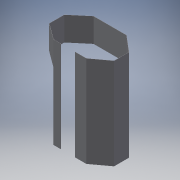
# Autodesk Inventor part: Main Cover
Saved by Autodesk Inventor 2016 (Build 200138000, 138)
## iProperties
Created: 2017-08-22
Part Number: Main Cover
Material: Generic
Document SubType Name: Modeling
Designer: m227586
Density: 1 g/cm^3
Appearance: Default
Author: m227586
Autodesk Inventor part; units mm, degrees
ref_plane "YZ Plane" through (0, 0, 0) normal (1, 0, 0) x (0, 1, 0)
ref_plane "XZ Plane" through (0, 0, 0) normal (0, 1, 0) x (-1, 0, 0)
sketch "Sketch2" plane through (0, 0, 0) normal (0, 0, 1) x (1, 0, 0)
  line L0 (7.8638, 351.0024) -> (-267.6362, 351.0024)
  line L1 (-267.6362, 351.0024) -> (-534, 125.5)
  line L2 (-534, 125.5) -> (-534, -125.5)
  line L3 (-534, -125.5) -> (-267.6362, -321.9976)
  line L4 (-267.6362, -321.9976) -> (7.8638, -321.9976)
  line L5 (7.8638, 351.0024) -> (7.8638, -321.9976) construction
  line L6 (-534, 0) -> (0, 0) construction
  line L7 (7.8638, 351.0024) -> (283.3638, 351.0024)
  line L8 (283.3638, 351.0024) -> (549.7276, 125.5)
  line L9 (549.7276, 125.5) -> (549.7276, -125.5)
  line L10 (549.7276, -125.5) -> (283.3638, -321.9976)
  line L11 (283.3638, -321.9976) -> (7.8638, -321.9976)
  dimension "d19" = 673
  dimension "d20" = 275.5
  dimension "d21" = 251
  dimension "d22" = 349
  dimension "d23" = 331
  dimension "d24" = 275.5
  dimension "d25" = 534
  constraints: 24 end point, 4 symmetric about line, 2 perpendicular, 2 vertical, 1 horizontal, 1 horizontal alignment, 1 midpoint
  measures "d19" distance of L0.start L4.end
  measures "d20" distance of L0.start L0.end
  measures "d21" distance of L1.end L2.end
  measures "d22" distance of L0.end L1.end
  measures "d23" distance of L2.end L3.end
  measures "d24" distance of L3.end L4.end
  measures "d25" distance of L6.start L6.end
ref_plane "Work Plane1" through (0, 0, 200) normal (0, 0, 1) x (1, 0, 0)
extrude "Extrusion1" add sketch "Sketch2" along normal blind 1306
shell "Shell2" thickness 3 removed faces 0
sketch "Sketch4" plane through (0, 0, 1306) normal (0, 0, 1) x (1, 0, 0)
  line L0 (-534, 125.5) -> (-267.6362, 351.0024)
  line L1 (-266.5368, 348.0024) -> (-531, 124.1091) projected
  line L2 (549.7276, 125.5) -> (283.3638, 351.0024) projected
  line L3 (-267.6362, 351.0024) -> (283.3638, 351.0024)
  line L4 (283.3638, 351.0024) -> (549.7276, 125.5)
  line L5 (546.7276, 124.1091) -> (282.2645, 348.0024) projected
  line L6 (283.3638, -321.9976) -> (549.7276, -125.5) projected
  line L7 (549.7276, 125.5) -> (549.7276, -125.5)
  line L8 (549.7276, -125.5) -> (283.3638, -321.9976)
  line L9 (-534, -125.5) -> (-267.6362, -321.9976) projected
  line L10 (283.3638, -321.9976) -> (-267.6362, -321.9976)
  line L11 (-534, 125.5) -> (-534, -125.5) projected
  line L12 (-267.6362, -321.9976) -> (-534, -125.5)
  line L13 (-534, -125.5) -> (-534, 125.5)
  line L14 (-531, 124.1091) -> (-531, -123.9851) projected
  point P0 (0, 0)
  constraints: 16 end point, 3 parallel, 2 collinear, 2 perpendicular, 1 horizontal
extrude "Extrusion2" cut sketch "Sketch4" against normal blind 3
sketch "Sketch5" plane through (0, 0, 0) normal (0, 0, -1) x (-1, 0, 0)
  line L0 (-283.3638, -321.9976) -> (-549.7276, -125.5) projected
  line L1 (-549.7276, 125.5) -> (-549.7276, -125.5)
  line L2 (-549.7276, -125.5) -> (-283.3638, -321.9976)
  line L3 (267.6362, -321.9976) -> (-283.3638, -321.9976) projected
  line L4 (-283.3638, -321.9976) -> (267.6362, -321.9976)
  line L5 (534, 125.5) -> (534, -125.5) projected
  line L6 (267.6362, -321.9976) -> (534, -125.5)
  line L7 (534, -125.5) -> (534, 125.5)
  line L8 (531, 124.1091) -> (531, -123.9851) projected
  line L9 (-283.3638, 351.0024) -> (267.6362, 351.0024) projected
  line L10 (534, 125.5) -> (267.6362, 351.0024)
  line L11 (267.6362, 351.0024) -> (-283.3638, 351.0024)
  line L12 (-549.7276, 125.5) -> (-283.3638, 351.0024) projected
  line L13 (-283.3638, 351.0024) -> (-549.7276, 125.5)
  point P0 (0, 0)
  constraints: 16 end point, 3 collinear, 2 parallel, 1 vertical
extrude "Extrusion3" cut sketch "Sketch5" against normal blind 3
sketch "Sketch6" plane through (-534, -125.5, 1303) normal (-1, 0, 0) x (0, 0, 1)
  line L0 (0, 251) -> (0, 476.5024) projected
  line L1 (0, 251) -> (-400, 251)
  line L2 (-1300, 251) -> (0, 251) projected
  line L3 (0, 251) -> (400, 251) construction
  line L4 (-400, 251) -> (-400, -196.4976)
  line L5 (-400, -196.4976) -> (-1300, -196.4976)
  line L6 (-1300, 473.5024) -> (0, 473.5024) projected
  line L7 (-400, 473.5024) -> (-400, 251)
  line L8 (-1300, 476.5024) -> (0, 476.5024) projected
  line L9 (-1300, -196.4976) -> (-1300, 476.5024)
  line L10 (-1300, 476.5024) -> (-400, 476.5024)
  line L11 (-400, 476.5024) -> (-400, 251)
  line L12 (-1300, 1.5149) -> (-1300, -193.4976) projected
  line L13 (-1300, -193.4976) -> (-400, -193.4976)
  line L14 (-1300, -193.4976) -> (0, -193.4976) projected
  point P0 (-1303, 125.5)
  dimension "d51" = 400
  dimension "d52" = 180
  constraints: 18 end point, 4 point on line, 3 collinear, 1 horizontal, 1 perpendicular, 1 vertical
  measures "d51" distance of L0.start L1.end
  measures "d52" angle of L1 L3
extrude "Extrusion4" cut sketch "Sketch6" against normal blind 816.377 contours L4 L13 L9 L2 | L2 L9 L6 L7 | L6 L9 L8 L11 | L4 L5 L9 L13
sketch "Sketch7" plane through (-534, -125.5, 903) normal (0, 0, -1) x (-1, 0, 0)
  line L0 (-3, 1.5149) -> (-267.3506, -193.4976) projected
  line L1 (-267.3506, -193.4976) -> (-267.3506, -196.4976)
  line L2 (-817.3638, -196.4976) -> (-266.3638, -196.4976) projected
  line L3 (-267.3506, -196.4976) -> (-389.3506, -196.4976)
  line L4 (-389.3506, -196.4976) -> (-389.3506, -193.4976)
  line L5 (-267.3506, -193.4976) -> (-816.377, -193.4976) projected
  line L6 (-389.3506, -193.4976) -> (-267.3506, -193.4976)
  line L7 (-267.3506, -193.4976) -> (-389.3506, -193.4976)
  point P0 (-534, 125.5)
  dimension "d55" = 122
  constraints: 10 end point, 3 point on line, 2 perpendicular, 1 collinear, 1 vertical
  measures "d55" distance of L1.end L3.end
extrude "Extrusion5" add sketch "Sketch7" along normal blind 900
sketch "Sketch8" plane through (283.3638, -321.9976, 903) normal (0, 0, -1) x (-1, 0, 0)
  line L0 (0, 0) -> (551, 0) projected
  line L1 (0.9868, 3) -> (190.9868, 3)
  line L2 (190.9868, 3) -> (190.9868, 0)
  line L3 (190.9868, 0) -> (0.9868, 0)
  line L4 (0.9868, 0) -> (0.9868, 3)
  point P0 (283.3638, 321.9976)
  dimension "d58" = 190
  constraints: 8 end point, 2 parallel, 1 horizontal, 1 perpendicular, 1 point on line
  measures "d58" distance of L2.end L3.end
extrude "Extrusion6" add sketch "Sketch8" along normal blind 900
sketch "Sketch9" plane through (-266.6494, -318.9976, 1303) normal (0, 1, 0) x (1, 0, 0)
  line L0 (359.0264, 400) -> (359.0264, 0)
  line L1 (0, 0) -> (549.0264, 0) projected
  line L2 (359.0264, 400) -> (359.0264, 1300) projected
  line L3 (359.0264, 0) -> (122, 0)
  line L4 (550.0132, 0) -> (-0.9868, 0) projected
  line L5 (122, 400) -> (122, 1300) projected
  line L6 (122, 0) -> (122, 400)
  line L7 (122, 400) -> (359.0264, 400) projected
  line L8 (359.0264, 400) -> (122, 400)
  point P0 (266.6494, 1303)
  constraints: 8 end point, 3 perpendicular, 2 point on line, 1 collinear
extrude "Extrusion7" cut sketch "Sketch9" against normal blind 3
sketch "Sketch10" plane through (0, 0, 3) normal (0, 0, -1) x (-1, 0, 0)
  line L0 (-283.3638, 351.0024) -> (-282.377, 351.0024)
  line L1 (-282.377, 347.9071) -> (-282.377, 351.0024) projected
  line L2 (-282.377, 351.0024) -> (-282.377, 347.9071)
  line L3 (-282.377, 347.9071) -> (-546.7276, 124.1091)
  line L4 (-546.7276, 124.1091) -> (-282.2645, 348.0024) projected
  line L5 (-282.377, -318.9976) -> (-546.7276, -123.9851) projected
  line L6 (-546.7276, 124.1091) -> (-546.7276, -123.9851)
  line L7 (-546.7276, -123.9851) -> (-282.377, -318.9976)
  line L8 (-92.377, -318.9976) -> (-282.377, -318.9976) projected
  line L9 (-282.377, -318.9976) -> (-92.377, -318.9976)
  line L10 (-92.377, -318.9976) -> (-92.377, -321.9976)
  line L11 (-282.377, -321.9976) -> (-283.3638, -321.9976) projected
  line L12 (-92.377, -321.9976) -> (-283.3638, -321.9976)
  line L13 (-283.3638, -321.9976) -> (-549.7276, -125.5) projected
  line L14 (-283.3638, -321.9976) -> (-549.7276, -125.5)
  line L15 (-549.7276, -125.5) -> (-549.7276, 125.5) projected
  line L16 (-549.7276, -125.5) -> (-549.7276, 125.5)
  line L17 (-549.7276, 125.5) -> (-283.3638, 351.0024)
  point P0 (0, 0)
  constraints: 22 end point, 7 collinear, 2 parallel, 1 horizontal, 1 perpendicular
extrude "Extrusion8" add sketch "Sketch10" along normal blind 225
sketch "Sketch11" plane through (-534, -125.5, 3) normal (0, 0, -1) x (-1, 0, 0)
  line L0 (-389.3506, -193.4976) -> (-389.3506, -196.4976) projected
  line L1 (-389.3506, -193.4976) -> (-389.3506, -196.4976)
  line L2 (-389.3506, -196.4976) -> (-267.3506, -196.4976) projected
  line L3 (-389.3506, -196.4976) -> (-267.3506, -196.4976)
  line L4 (-267.3506, -193.4976) -> (-389.3506, -193.4976) projected
  line L5 (-267.3506, -196.4976) -> (-267.3506, -193.4976)
  line L6 (-267.3506, -193.4976) -> (-389.3506, -193.4976)
  point P0 (-534, 125.5)
  constraints: 8 end point, 2 equal length, 1 perpendicular, 1 vertical
extrude "Extrusion9" add sketch "Sketch11" along normal blind 225
sketch "Sketch12" plane through (282.377, -318.9976, 1303) normal (0, 1, 0) x (1, 0, 0)
  line L0 (-190, 0) -> (-190, 1525) projected
  line L1 (-190, 1300) -> (-190, 0) projected
  line L2 (-190, 1525) -> (-190, 0)
  line L3 (-190, 0) -> (-188.679, 0)
  line L4 (-550.0132, 0) -> (0.9868, 0) projected
  line L5 (-188.679, 0) -> (-188.679, 1525)
  line L6 (-190, 1525) -> (0, 1525) projected
  line L7 (-188.679, 1525) -> (-190, 1525)
  point P0 (-282.377, 1303)
  dimension "d67" = 1.321
  constraints: 8 end point, 2 collinear, 2 point on line, 1 perpendicular
  measures "d67" distance of L0.start L3.end
extrude "Extrusion10" cut sketch "Sketch12" against normal blind 3
sketch "Sketch15" plane through (282.377, -318.9976, 3) normal (0, 1, 0) x (1, 0, 0)
  line L0 (0, -900) -> (0, 225) projected
  line L1 (0, 225) -> (0, 202)
  line L2 (-188.679, -1300) -> (-188.679, 225) projected
  line L3 (-188.679, 225) -> (-188.679, 202)
  line L4 (-188.679, 202) -> (-21.679, 202)
  line L5 (-21.679, 202) -> (-21.679, 225)
  line L6 (-188.679, 225) -> (0, 225) projected
  line L7 (-21.679, 225) -> (-188.679, 225)
  circle A0 centre (-41.679, 213.5) radius 5
  circle A1 centre (-168.679, 213.5) radius 5
  point P0 (-282.377, 3)
  dimension "d95" = 23
  dimension "d97" = 167
  dimension "d98" = 10
  dimension "d99" = 10
  dimension "d100" = 20
  dimension "d101" = 20
  constraints: 10 end point, 3 point on line, 2 centre point, 2 perpendicular, 1 collinear
  measures "d95" distance of L0.end L1.end
  measures "d97" distance of L3.end L4.end
  measures "d98" diameter of A0
  measures "d99" diameter of A1
  measures "d100" distance from line of L2 A1.centre
  measures "d101" distance from line of L5 A0.centre
extrude "Extrusion11" cut sketch "Sketch15" against normal blind 3 contours A0 | A1
body "Solid2"
